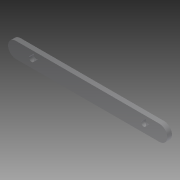
# Autodesk Inventor part: Handle
Saved by Autodesk Inventor 2015 (Build 190159000, 159)
## iProperties
Created: 2016-11-22
Part Number: Handle
Material: Polycarbonate, Clear
Document SubType Name: Modeling
Designer: James Yelland
Density: 1.2 g/cm^3
Appearance: Polycarbonate - Clear
Author: James Yelland
Autodesk Inventor part; units mm, degrees
ref_plane "YZ Plane" through (0, 0, 0) normal (1, 0, 0) x (0, 1, 0)
ref_plane "XZ Plane" through (0, 0, 0) normal (0, 1, 0) x (-1, 0, 0)
ref_plane "XY Plane" through (0, 0, 0) normal (0, 0, 1) x (1, 0, 0)
sketch "Sketch1" plane through (0, 0, 0) normal (0, 1, 0) x (-1, 0, 0)
  circle A0 centre (-35.5968, 0) radius 1.6
  circle A1 centre (35.5968, 0) radius 1.6
  line L0 (50.5968, 0) -> (50.5968, 0)
  line L1 (-50.5968, 0) -> (-50.5968, 0)
  line L2 (-45.5968, -5) -> (45.5968, -5)
  line L3 (50.5968, 0) -> (50.5968, 0)
  line L4 (45.5968, 5) -> (-45.5968, 5)
  line L5 (-50.5968, 0) -> (-50.5968, 0)
  arc A2 (50.5968, 0) -> (45.5968, 5) centre (45.5968, 0) ccw
  arc A3 (45.5968, -5) -> (50.5968, 0) centre (45.5968, 0) ccw
  arc A4 (-45.5968, 5) -> (-50.5968, 0) centre (-45.5968, 0) ccw
  arc A5 (-50.5968, 0) -> (-45.5968, -5) centre (-45.5968, 0) ccw
  point P0 (50.5968, -5)
  point P1 (-50.5968, -5)
  dimension "d6" = 5
  dimension "d7" = 15
  dimension "d10" = 5
  constraints: 12 end point, 8 point on circle, 8 tangent, 6 centre point, 4 point on line, 3 equal radius, 3 perpendicular, 1 vertical
  measures "d6" distance of L0.start point (50.597, -5)
  measures "d7" distance of A0.centre L1.start
  measures "d10" radius of A2
extrude "Extrusion1" add sketch "Sketch1" along normal blind 3
body "Solid1"
